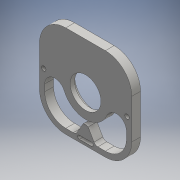
# Autodesk Inventor part: Del 6
Saved by Autodesk Inventor 2016 (Build 200138000, 138)
## iProperties
Created: 2017-01-26
Part Number: Del 6
Material: Generic
Document SubType Name: Modeling
Designer: 16rasa
Density: 1 g/cm^3
Appearance: Default
Author: 16rasa
Autodesk Inventor part; units mm, degrees
ref_plane "YZ Plane" through (0, 0, 0) normal (1, 0, 0) x (0, 1, 0)
ref_plane "XZ Plane" through (0, 0, 0) normal (0, 1, 0) x (-1, 0, 0)
ref_plane "XY Plane" through (0, 0, 0) normal (0, 0, 1) x (1, 0, 0)
sketch "Sketch1" plane through (0, 0, 0) normal (0, 1, 0) x (-1, 0, 0)
  line L0 (52.5, 52.5) -> (-52.5, 52.5)
  line L1 (-52.5, 52.5) -> (-52.5, -52.5)
  line L2 (-52.5, -52.5) -> (52.5, -52.5)
  line L3 (52.5, -52.5) -> (52.5, 52.5)
  line L4 (52.5, 52.5) -> (-52.5, -52.5) construction
  line L5 (-52.5, 52.5) -> (52.5, -52.5) construction
  point P0 (0, 0)
  dimension "d0" = 105
  dimension "d1" = 105
  constraints: 12 end point, 2 midpoint, 2 parallel, 1 horizontal, 1 perpendicular
  measures "d0" distance of L2.end L1.end
  measures "d1" distance of L1.end L0.end
extrude "Extrusion1" add sketch "Sketch1" along normal blind 10
fillet "Fillet1" radius 30 4 edges at (-52.5, 5, -52.5) (-52.5, 5, 52.5) (52.5, 5, -52.5) (52.5, 5, 52.5)
sketch "Sketch2" plane through (0, 10, 0) normal (0, 1, 0) x (1, 0, 0)
  circle A0 centre (0, 0) radius 17.5
  dimension "d5" = 35
  constraints: 1 centre point, 1 coincident
  measures "d5" diameter of A0
extrude "Extrusion2" cut sketch "Sketch2" against normal blind 10
chamfer "Chamfer1" distance 5 angle 45 1 edges at (-17.5, 10, 0)
sketch "Sketch3" plane through (0, 10, 0) normal (0, 1, 0) x (1, 0, 0)
  arc A0 (22.5, -52.5) -> (52.5, -22.5) centre (22.5, -22.5) ccw projected
  line L0 (52.5, -22.5) -> (52.5, 22.5) projected
  arc A1 (52.5, 22.5) -> (22.5, 52.5) centre (22.5, 22.5) ccw projected
  line L1 (22.5, 52.5) -> (-22.5, 52.5) projected
  arc A2 (-22.5, 52.5) -> (-52.5, 22.5) centre (-22.5, 22.5) ccw projected
  line L2 (-52.5, 22.5) -> (-52.5, -22.5) projected
  arc A3 (-52.5, -22.5) -> (-22.5, -52.5) centre (-22.5, -22.5) ccw projected
  line L3 (-22.5, -52.5) -> (22.5, -52.5) projected
  circle A4 centre (0, 0) radius 22.5 projected
  line L4 (46.5, 22.5) -> (46.5, -22.5)
  arc A5 (22.5, -46.5) -> (46.5, -22.5) centre (22.5, -22.5) ccw
  line L5 (22.5, -46.5) -> (-22.5, -46.5)
  arc A6 (-46.5, -22.5) -> (-22.5, -46.5) centre (-22.5, -22.5) ccw
  line L6 (-46.5, -22.5) -> (-46.5, 22.5)
  arc A7 (-22.5, 46.5) -> (-46.5, 22.5) centre (-22.5, 22.5) ccw
  line L7 (-22.5, 46.5) -> (22.5, 46.5)
  arc A8 (46.5, 22.5) -> (22.5, 46.5) centre (22.5, 22.5) ccw
  circle A9 centre (0, 0) radius 26.5
  arc A10 (24.4079, 10.3201) -> (46.5, 14.7986) centre (35, 14.7986) ccw
  arc A11 (-46.5, 14.7986) -> (-24.4079, 10.3201) centre (-35, 14.7986) ccw
  dimension "d11" = 6
  dimension "d12" = 4
  dimension "d13" = 23
  dimension "d14" = 23
  constraints: 14 point on circle, 8 end point, 7 centre point, 4 tangent, 2 point on line, 7 other
  measures "d11" distance between parallel lines of L0 L4
  measures "d12" radial gap between concentric circles of A4 A9
  measures "d13" diameter of A10
  measures "d14" diameter of A11
extrude "Extrusion3" cut sketch "Sketch3" against normal blind 10 contours L4 A10 A9 A11 L6 A7 L7 A8
sketch "Sketch5" plane through (0, 10, 0) normal (0, 1, 0) x (1, 0, 0)
  line L0 (52.2088, 0) -> (47.2088, 0)
  line L1 (-52.5, 22.5) -> (-52.5, -22.5) projected
  line L2 (-52.5, 0) -> (-47.5, 0)
  circle A0 centre (47.2088, 0) radius 2.5
  circle A1 centre (-47.5, 0) radius 2.5
  point P0 (0, 0)
  dimension "d21" = 5
  dimension "d22" = 5
  dimension "d23" = 5
  dimension "d24" = 5
  constraints: 4 end point, 2 centre point, 2 coincident, 2 horizontal, 1 midpoint
  measures "d21" distance of L0.start L0.end
  measures "d22" distance of L2.start L2.end
  measures "d23" diameter of A0
  measures "d24" diameter of A1
extrude "Extrusion4" cut sketch "Sketch5" against normal blind 10
sketch "Sketch6" plane through (0, 10, 0) normal (0, 1, 0) x (1, 0, 0)
  line L0 (52.5, 52.5) -> (14.5, 52.5)
  line L1 (22.5, 52.5) -> (-22.5, 52.5) projected
  line L2 (-52.5, 52.5) -> (-14.5, 52.5)
  line L3 (0, 52.5) -> (0, 31.5)
  line L4 (0, 31.5) -> (0, 37)
  arc A0 (-5.4968, 36.8121) -> (5.4968, 36.8121) centre (0, 37) ccw
  line L5 (14.5, 52.5) -> (2.9353, 32.3488)
  line L6 (-2.9353, 32.3488) -> (-14.5, 52.5)
  point P0 (0, 0)
  dimension "d27" = 38
  dimension "d28" = 38
  dimension "d29" = 21
  dimension "d30" = 5.5
  dimension "d31" = 11
  constraints: 12 end point, 5 point on line, 4 point on circle, 1 centre point, 1 coincident, 1 midpoint, 1 vertical
  measures "d27" distance of L0.start L0.end
  measures "d28" distance of L2.start L2.end
  measures "d29" distance of L3.start L3.end
  measures "d30" distance of L3.end L4.end
  measures "d31" diameter of A0
extrude "Extrusion5" add sketch "Sketch6" against normal blind 10 contours L5 A0 L3 L1 | L3 A0 L6 L1
fillet "Fillet2" radius 5 2 edges at (11.0566, 5, -46.5) (-11.0566, 5, -46.5)
sketch "Sketch7" plane through (0, 10, 0) normal (0, 1, 0) x (1, 0, 0)
  line L0 (22.5, 52.5) -> (-22.5, 52.5) projected
  line L1 (0, 47.5) -> (-7, 47.5)
  line L2 (-7, 47.5) -> (7, 47.5)
  arc A0 (7, 45.5) -> (7, 49.5) centre (7, 47.5) ccw
  arc A1 (-7, 49.5) -> (-7, 45.5) centre (-7, 47.5) ccw
  line L3 (7, 45.5) -> (-7, 45.5)
  line L4 (-7, 49.5) -> (7, 49.5)
  point P0 (0, 0)
  dimension "d37" = 14
  dimension "d38" = 4
  dimension "d39" = 4
  constraints: 8 end point, 4 point on circle, 3 tangent, 2 centre point, 2 coincident, 1 point on line
  measures "d37" distance of L1.end L2.end
  measures "d38" diameter of A0
  measures "d39" diameter of A1
extrude "Extrusion6" cut sketch "Sketch7" against normal blind 10
body "Solid1"
